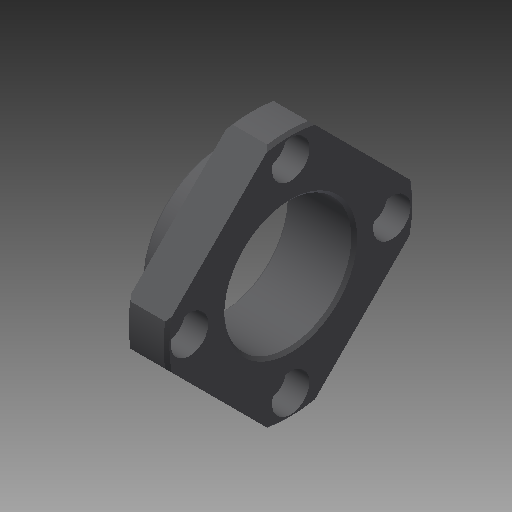
# Autodesk Inventor part: FF 10Part1
Saved by Autodesk Inventor 2018 (Build 220112000, 112)
## iProperties
Category: PARTsolutions
Company: THK
Created: 2017-06-20
Part Number: FF 10Part1
Catalog Web Link: www.cadenas.de
Description: Supported side type FF-P1-
Vendor: THK
Document SubType Name: Modeling
Designer: psAdmin
Manufacturer: THK
Mass: 6.10505 g
Surface Area: 40.5619 cm^2
Volume: 6.10505 cm^3
Density: 1 g/cm^3
Material: Generic
Appearance: PSOLRGB-192-192-192
PSOL_IDENT_0: {$CADENAS_DATA\23d-libs\thk\fed_screw\ball_screw\ball_screw_peripheral\suport_unit\supported_ff_1.pr
PSOL_IDENT_1: j},181 {VTYP=3D},{NB=FF 10Part1},{LINA=FF 10Part1},{NN=Supported side type FF-P1},{DATE=02.06.2017 0
PSOL_IDENT_2: 6:41:21},{GEOMDATE=23.05.2016 06:26:00},{VERSION=},{LINEID=50},{LINESUBID=-1},{WBVAR=}  {NB=FF 10Par
PSOL_IDENT_3: t1},{LINA=FF 10Part1},{KT=DUMMY},{IDNR=},{MN=FF 10},{SD=8.000},{L=12.000},{H=7.000},{F=5.000},{D=28.
PSOL_IDENT_4: 000},{A=43.000},{PCD=35.000},{B=35.000},{SD1=3.400},{SD2=6.500},{SH=4.000},{T=16.000},{TX=19.000},{T
PSOL_IDENT_5: Y=15.000},{SYL=21.000},{SD4=12.000},{DX=9.500},{DY=8.000},{DB=20.000},{L4=1.000},{DW=22.000},{SDX=22
PSOL_IDENT_6: .000}
NN: Supported side type FF-P1
NB: FF 10Part1
NBSYN: $MN.Part1
LINA: FF 10Part1
MN: FF 10
SD: 8.000
L: 12.000
H: 7.000
F: 5.000
D: 28.000
A: 43.000
PCD: 35.000
B: 35.000
SD1: 3.400
SD2: 6.500
SH: 4.000
T: 16.000
TX: 19.000
TY: 15.000
SYL: 21.000
SD4: 12.000
DX: 9.500
DY: 8.000
DB: 20.000
L4: 1.000
DW: 22.000
SDX: 22.000
SUPPLIER: THK
ARTICLENO: FF 10Part1
BOMINFO: FF 10Part1
CREATOR: CADENAS GmbH
Title: FF 10Part1
Author: Cadenas PARTsolutions
Autodesk Inventor part; units mm, degrees
ref_plane "YZ Plane" through (0, 0, 0) normal (1, 0, 0) x (0, 1, 0)
ref_plane "XZ Plane" through (0, 0, 0) normal (0, 1, 0) x (-1, 0, 0)
ref_plane "XY Plane" through (0, 0, 0) normal (0, 0, 1) x (1, 0, 0)
sketch "Sketch_1" plane through (0, 0, 0) normal (0, 0, 1) x (1, 0, 0)
  line L0 (50, 0) -> (-50, 0)
  line L1 (-5, 11.5) -> (-4.5, 11)
  line L2 (-4.5, 11) -> (6.5, 11)
  line L3 (6.5, 11) -> (7, 11.5)
  line L4 (7, 11.5) -> (7, 21)
  line L5 (7, 21) -> (6.5, 21.5)
  line L6 (6.5, 21.5) -> (0.5, 21.5)
  line L7 (0.5, 21.5) -> (0, 21)
  line L8 (0, 21) -> (0, 14.25)
  arc A0 (-0.25, 14) -> (0, 14.25) centre (-0.25, 14.25) ccw
  line L9 (-0.25, 14) -> (-4.5, 14)
  line L10 (-4.5, 14) -> (-5, 13.5)
  line L11 (-5, 13.5) -> (-5, 11.5)
  constraints: 24 end point, 2 point on circle, 1 centre point
revolve "Revolution1" add sketch "Sketch_1" angle 360 about axis through (50, 0, 0) along (1, 0, 0)
sketch "Sketch_2" plane through (7, 0, 0) normal (1, 0, 0) x (0, 0, -1)
  line L0 (-49.4975, 0) -> (0, -49.4975)
  line L1 (0, -49.4975) -> (49.4975, 0)
  line L2 (49.4975, 0) -> (0, 49.4975)
  line L3 (0, 49.4975) -> (-49.4975, 0)
  line L4 (-24.7487, 0) -> (0, -24.7487)
  line L5 (0, -24.7487) -> (24.7487, 0)
  line L6 (24.7487, 0) -> (0, 24.7487)
  line L7 (0, 24.7487) -> (-24.7487, 0)
  constraints: 16 end point
extrude "Extrusion1" cut sketch "Sketch_2" against normal blind 7
sketch "Sketch3" plane through (7, 0, 0) normal (1, 0, 0) x (0, 0, -1)
  point P0 (0, 17.5)
hole "Hole1" at (7, 17.5, 0) direction (-1, 0, 0) diameter 3.4 depth 7 counterbore diameter 6.5 counterbore depth 4
pattern_linear "Rectangular Pattern1" count 2 spacing 24.7487 along (0, -0.7071068, 0.7071068) count 2 spacing 24.7487 along (0, -0.7071068, -0.7071068) of "Hole1"
ref_plane "ff_1_XY" through (0, 0, 0) normal (1, 0, 0) x (0, 0, -1)
ref_plane "ff_1_YZ" through (0, 0, 0) normal (0, 0, -1) x (0, 1, 0)
ref_plane "ff_1_ZX" through (0, 0, 0) normal (0, 1, 0) x (1, 0, 0)
ref_plane "ff_2x_XY" through (1, 0, 0) normal (1, 0, 0) x (0, 0, -1)
ref_plane "ff_2x_YZ" through (1, 0, 0) normal (0, 0, -1) x (0, 1, 0)
ref_plane "ff_2x_ZX" through (1, 0, 0) normal (0, 1, 0) x (1, 0, 0)
body "Solid1"
